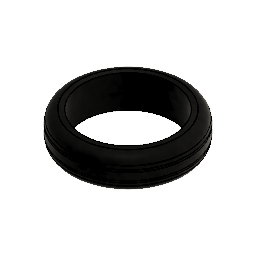
tire v4 (Autodesk Fusion 360 design; units mm, degrees)
Autodesk Fusion 360 part; units mm, degrees
sketch "スケッチ1" plane through (0, 0, 0) normal (0, 1, 0) x (1, 0, 0)
  line L0 (0, 0) -> (4.8, 0)
  line L1 (4.8, 0) -> (4.8, -3.5)
  line L2 (4.8, -3.5) -> (6.15, -3.5)
  line L3 (6.15, -3.5) -> (6.4, -2.25)
  line L4 (6.4, -2.25) -> (6.4, -1.25)
  line L5 (6.4, -1.25) -> (6.15, 0)
  line L6 (6.15, 0) -> (4.8, 0)
  dimension "d1" = 3.5
  dimension "d3" = 4.8
  dimension "d4" = 1
  dimension "d5" = 0.25
  dimension "d8" = 6.4
  measures "d3" distance of L0.start
  measures "d8" distance of L0.start L4
revolve "回転1" add sketch "スケッチ1" angle 360 about axis through (0, 0, 1.75) along (0, 0, 1)
fillet "フィレット1" radius 1 4 edges at (-5.7338, -2.2239, 0) (-5.9669, -2.3143, 1.25) (-5.9669, -2.3143, 2.25) (-5.7338, -2.2239, 3.5)
equation "d8 = ( 12.8 / 2 ) * 1 mm"
